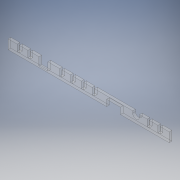
# Autodesk Inventor part: Back
Saved by Autodesk Inventor 2017 (Build 210142000, 142)
## iProperties
Created: 2017-04-17
Part Number: Back
Material: Generic
Document SubType Name: Modeling
Designer: jeffkub
Density: 1 g/cm^3
Appearance: Polycarbonate - Clear
Author: jeffkub
Autodesk Inventor part; units mm, degrees
ref_plane "YZ Plane" through (0, 0, 0) normal (1, 0, 0) x (0, 1, 0)
ref_plane "XZ Plane" through (0, 0, 0) normal (0, 1, 0) x (-1, 0, 0)
ref_plane "XY Plane" through (0, 0, 0) normal (0, 0, 1) x (1, 0, 0)
sketch "Sketch1" plane through (0, 0, 0) normal (0, 0, 1) x (1, 0, 0)
  line L0 (89.1, -5.2) -> (-89.1, -5.2)
  line L1 (-89.1, -5.2) -> (-89.1, 5.2)
  line L2 (-89.1, 5.2) -> (89.1, 5.2)
  line L3 (89.1, 5.2) -> (89.1, -5.2)
  line L4 (89.1, -5.2) -> (-89.1, 5.2) construction
  line L5 (-89.1, -5.2) -> (89.1, 5.2) construction
  point P0 (0, 0)
  dimension "d0" = 10.4
  dimension "d1" = 178.2
  constraints: 12 end point, 2 midpoint, 2 parallel, 1 horizontal, 1 perpendicular
  measures "d0" distance of L2.end L0.start
  measures "d1" distance of L1.end L2.end
extrude "Extrusion1" add sketch "Sketch1" along normal blind 3
sketch "Sketch2" plane through (0, 0, 0) normal (0, 0, -1) x (-1, 0, 0)
  line L0 (-89.1, -5.2) -> (89.1, -5.2) projected
  line L1 (45.1, 5.2) -> (54.9, 5.2)
  line L2 (54.9, 5.2) -> (54.9, -3.7)
  line L3 (54.9, -3.7) -> (45.1, -3.7)
  line L4 (45.1, -3.7) -> (45.1, 5.2)
  line L5 (89.1, 5.2) -> (-89.1, 5.2) projected
  arc A0 (-56.275, 3) -> (-48.725, 3) centre (-52.5, 3) ccw
  line L6 (-56.275, 3) -> (-56.275, 5.2)
  line L7 (-48.725, 3) -> (-48.725, 5.2)
  line L8 (-56.275, 5.2) -> (-48.725, 5.2)
  arc A1 (-48.725, 3) -> (-56.275, 3) centre (-52.5, 3) ccw construction
  line L9 (-35.1, 1.8) -> (-19.9, 1.8)
  line L10 (-19.9, 1.8) -> (-19.9, -5.2)
  line L11 (-19.9, -5.2) -> (-35.1, -5.2)
  line L12 (-35.1, -5.2) -> (-35.1, 1.8)
  line L13 (89.1, -5.2) -> (-89.1, -5.2) projected
  point P0 (0, 0)
  point P1 (50, 2.9)
  point P2 (50, 5.2)
  point P3 (-27.5, -2.25)
  point P4 (-27.5, 1.8)
  dimension "d4" = 50
  dimension "d5" = 8.1
  dimension "d6" = 1.5
  dimension "d7" = 9.8
  dimension "d8" = 52.5
  dimension "d9" = 7.55
  dimension "d10" = 8.2
  dimension "d13" = 27.5
  dimension "d14" = 2.95
  dimension "d16" = 7
  dimension "d17" = 15.2
  constraints: 22 end point, 4 parallel, 4 point on circle, 3 collinear, 2 centre point, 2 horizontal, 2 midpoint, 2 perpendicular, 2 point on line, 2 tangent, 2 vertical, 2 vertical alignment
  measures "d4" horizontal distance of point (50, 2.9) point (0, 0)
  measures "d5" distance from line of L0 point (50, 2.9)
  measures "d6" distance between parallel lines of L0 L3
  measures "d7" distance of L1.start L1.end
  measures "d8" horizontal distance of point (0, 0) A0.centre
  measures "d9" diameter of A0
  measures "d10" distance from line of L0 A0.centre
  measures "d13" horizontal distance of point (-27.5, -2.25) point (0, 0)
  measures "d14" distance from line of L0 point (-27.5, -2.25)
  measures "d16" distance of L11.end L9.start
  measures "d17" distance of L9.start L9.end
extrude "Extrusion2" cut sketch "Sketch2" against normal through all
sketch "Sketch3" plane through (0, 0, 0) normal (0, 0, -1) x (-1, 0, 0)
  line L0 (-56.275, 5.2) -> (-89.1, 5.2) projected
  line L1 (45.1, 5.2) -> (-48.725, 5.2) projected
  line L2 (89.1, 5.2) -> (54.9, 5.2) projected
  line L3 (-79.1, 5.2) -> (-76.6, 5.2)
  line L4 (-76.6, 5.2) -> (-76.6, -1.8)
  line L5 (-76.6, -1.8) -> (-79.1, -1.8)
  line L6 (-79.1, -1.8) -> (-79.1, 5.2)
  line L7 (-67.1, 5.2) -> (-64.6, 5.2)
  line L8 (-64.6, 5.2) -> (-64.6, -1.8)
  line L9 (-64.6, -1.8) -> (-67.1, -1.8)
  line L10 (-67.1, -1.8) -> (-67.1, 5.2)
  line L11 (-89.1, 5.2) -> (-89.1, -5.2) projected
  line L12 (64.6, 5.2) -> (67.1, 5.2)
  line L13 (67.1, 5.2) -> (67.1, -1.8)
  line L14 (67.1, -1.8) -> (64.6, -1.8)
  line L15 (64.6, -1.8) -> (64.6, 5.2)
  line L16 (76.6, 5.2) -> (79.1, 5.2)
  line L17 (79.1, 5.2) -> (79.1, -1.8)
  line L18 (79.1, -1.8) -> (76.6, -1.8)
  line L19 (76.6, -1.8) -> (76.6, 5.2)
  line L20 (89.1, -5.2) -> (89.1, 5.2) projected
  line L21 (32.1, 5.2) -> (29.6, 5.2)
  line L22 (29.6, 5.2) -> (29.6, -1.8)
  line L23 (29.6, -1.8) -> (32.1, -1.8)
  line L24 (32.1, -1.8) -> (32.1, 5.2)
  line L25 (20.1, 5.2) -> (17.6, 5.2)
  line L26 (17.6, 5.2) -> (17.6, -1.8)
  line L27 (17.6, -1.8) -> (20.1, -1.8)
  line L28 (20.1, -1.8) -> (20.1, 5.2)
  line L29 (8.1, 5.2) -> (5.6, 5.2)
  line L30 (5.6, 5.2) -> (5.6, -1.8)
  line L31 (5.6, -1.8) -> (8.1, -1.8)
  line L32 (8.1, -1.8) -> (8.1, 5.2)
  line L33 (-3.9, 5.2) -> (-6.4, 5.2)
  line L34 (-6.4, 5.2) -> (-6.4, -1.8)
  line L35 (-6.4, -1.8) -> (-3.9, -1.8)
  line L36 (-3.9, -1.8) -> (-3.9, 5.2)
  point P0 (0, 0)
  dimension "d18" = 2.5
  dimension "d19" = 10
  dimension "d21" = 7
  dimension "d24" = 12
  dimension "d25" = 10
  dimension "d26" = 12
  dimension "d28" = 12
  dimension "d29" = 12
  dimension "d30" = 35
  dimension "d31" = 12
  constraints: 64 end point, 19 collinear, 16 parallel, 8 horizontal, 8 perpendicular, 3 point on line
  measures "d18" distance of L4.end L5.end
  measures "d19" distance between parallel lines of L6 L11
  measures "d21" distance of L5.end L3.start
  measures "d24" distance between parallel lines of L10 L6
  measures "d25" distance between parallel lines of L17 L20
  measures "d26" distance between parallel lines of L13 L17
  measures "d28" distance between parallel lines of L32 L28
  measures "d29" distance between parallel lines of L36 L32
  measures "d30" distance between parallel lines of L24 L13
  measures "d31" distance between parallel lines of L24 L28
extrude "Extrusion3" cut sketch "Sketch3" against normal through all
equation "\"d26\" = d24"
equation "\"d28\" = d31"
equation "\"d29\" = d31"
equation "\"d31\" = d24"
body "Solid1"
